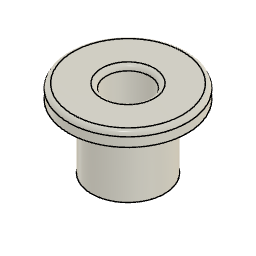
Leg_BearingMount_x24 (Autodesk Fusion 360 design; units mm, degrees)
Autodesk Fusion 360 part; units mm, degrees
sketch "Sketch1" plane through (0, 0, 0) normal (0, 0, 1) x (1, 0, 0)
  circle A0 centre (0, 0) radius 4
  dimension "d1" = 8
  constraint coincident A0.centre origin
  measures "d1" diameter of A0
extrude "Extrude1" add sketch "Sketch1" along normal blind 8
sketch "Sketch2" plane through (0, 0, 8) normal (0, 0, 1) x (-1, 0, 0)
  circle A0 centre (0, 0) radius 4
  circle A1 centre (0, 0) radius 2.375
  dimension "d4" = 4.75
  constraint coincident A0.centre A1.centre
  measures "d4" diameter of A1
extrude "Extrude2" cut sketch "Sketch2" against normal blind 3 contours A1
sketch "Sketch3" plane through (0, 0, 5) normal (0, 0, 1) x (-1, 0, 0)
  circle A0 centre (0, 0) radius 2.375
  circle A1 centre (0, 0) radius 1.5
  dimension "d7" = 3
  constraint concentric A0 A1
  measures "d7" diameter of A1
extrude "Extrude3" cut sketch "Sketch3" against normal blind 9 contours A1
sketch "Sketch4" plane through (0, 0, 8) normal (0, 0, 1) x (-1, 0, 0)
  circle A0 centre (0, 0) radius 2.375
  circle A1 centre (0, 0) radius 4
  circle A2 centre (0, 0) radius 6.5
  dimension "d10" = 13
  constraint coincident A0.centre A1.centre
  measures "d10" diameter of A2
extrude "Extrude4" add sketch "Sketch4" against normal blind 2 contours A2
extrude "Extrude5" add 1 faces at (3.1462, -0.2732, 0) along direction (0, 0, -1) blind 2
sketch "Sketch5" plane through (0, 0, -2) normal (0, 0, -1) x (1, 0, 0)
  circle A0 centre (0, 0) radius 1.5
  circle A1 centre (0, 0) radius 4
  circle A2 centre (0, 0) radius 3.2
  dimension "d18" = 6.4
  constraint concentric A0 A2
  measures "d18" diameter of A2
extrude "Extrude6" cut sketch "Sketch5" against normal blind 0.5 contours A1
extrude "Extrude7" add 1 faces at (2.6214, 0.159, -2) along direction (0, 0, -1) blind 0.5
extrude "Extrude8" add 1 faces at (3.7184, 0.1987, -1.5) along direction (0, 0, -1) blind 0.5
extrude "Extrude9" cut 1 faces at (-2.0745, 0.118, 5) along direction (0, 0, -1) blind 3
extrude "Extrude10" cut 1 faces at (-2.0745, 0.118, 2) along direction (0, 0, -1) blind 1.5
extrude "Extrude11" add 1 faces at (3.7184, 0.1987, -2) along direction (0, 0, -1) blind 0.5
chamfer "Chamfer3" distance 0.43 angle 45 2 edges at (1.3985, 0.5424, 0.5) (2.2143, -0.8588, 0.5)
extrude "Extrude12" cut 1 faces at (3.1462, 0.2732, -2.5) along direction (0, 0, 1) blind 1.5
extrude "Extrude13" cut 1 faces at (-5.092, 0.4409, 8) along direction (0, 0, -1) blind 0.5
fillet "Fillet2" radius 0.5 2 edges at (2.2143, 0.8588, 7.5) (6.0601, -2.3505, 7.5)
